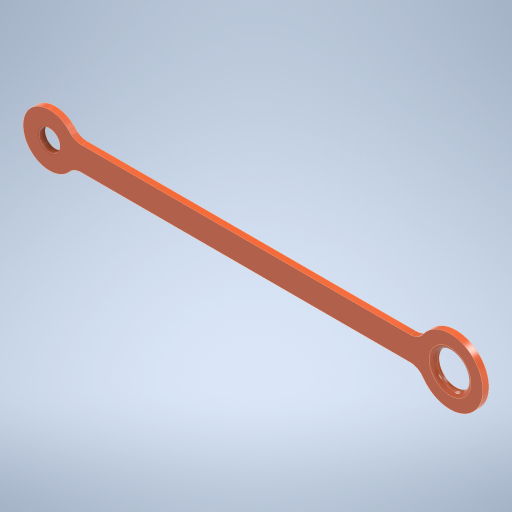
# Autodesk Inventor part: destek bağlantısı
Saved by Autodesk Inventor 2023.2 (Build 272271000, 271)
## iProperties
Created: 2022-12-25
Part Number: destek bağlantısı
Material: Polystyrene
Document SubType Name: Modeling
Designer: omrfrkmll
Density: 1.021 g/cm^3
Appearance: Smooth - Light Orange
Author: omrfrkmll
Autodesk Inventor part; units mm, degrees
ref_plane "YZ Plane" through (0, 0, 0) normal (1, 0, 0) x (0, 1, 0)
ref_plane "XZ Plane" through (0, 0, 0) normal (0, 1, 0) x (-1, 0, 0)
ref_plane "XY Plane" through (0, 0, 0) normal (0, 0, 1) x (1, 0, 0)
sketch "Sketch1" plane through (0, 0, 0) normal (0, 0, 1) x (1, 0, 0)
  line L0 (0, 0) -> (-34.0118, 0)
  line L1 (0, 0) -> (0, 29.864)
  circle A0 centre (-101.344, 0) radius 5.25
  arc A1 (-91.3761, 8.7294) -> (-91.3761, -8.7294) centre (-101.344, 0) ccw
  arc A2 (86.7622, -9.4286) -> (86.7622, 9.4286) centre (100.303, 0) ccw
  line L2 (-85.3577, 6) -> (80.197, 6)
  line L3 (-85.3577, -6) -> (80.197, -6)
  arc A3 (-91.3761, 8.7294) -> (-85.3577, 6) centre (-85.3577, 14) ccw
  arc A4 (-85.3577, -6) -> (-91.3761, -8.7294) centre (-85.3577, -14) ccw
  arc A5 (80.197, 6) -> (86.7622, 9.4286) centre (80.197, 14) ccw
  arc A6 (86.7622, -9.4286) -> (80.197, -6) centre (80.197, -14) ccw
  circle A7 centre (100.303, 0) radius 8.5
  point P0 (-89.5303, 6)
  point P1 (84.9326, 6)
  point P2 (-89.5303, -6)
  point P3 (84.9326, -6)
  dimension "d0" = 201.647
  dimension "d1" = 10.5
  dimension "d2" = 8
  dimension "d4" = 12
  dimension "d5" = 8
  dimension "d9" = 17
  dimension "d10" = 8
  constraints: 16 point on circle, 8 centre point, 8 end point, 8 tangent, 4 point on line, 3 equal radius, 2 horizontal, 2 symmetric about line, 1 coincident, 1 vertical
  measures "d0" distance of A2.centre A0.centre
  measures "d1" diameter of A0
  measures "d2" radial gap between concentric circles of A0 A1
  measures "d4" distance between parallel lines of L3 L2
  measures "d5" radius of A3
  measures "d9" diameter of A7
  measures "d10" radial gap between concentric circles of A2 A7
extrude "Extrusion1" add sketch "Sketch1" along normal blind 3
fillet "Fillet1" radius 2 1 edges at (91.803, 0, 3)
body "Solid1"
